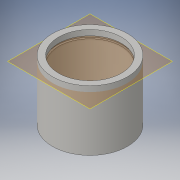
# Autodesk Inventor part: upper_arm_002
Saved by Autodesk Inventor 2016 SP1 (Build 200210100, 210)
## iProperties
Created: 2016-06-15
Part Number: upper_arm_002
Material: Generic
Document SubType Name: Modeling
Designer: asvsf
Density: 1 g/cm^3
Appearance: Default
Author: asvsf
Autodesk Inventor part; units mm, degrees
ref_plane "YZ Plane" through (0, 0, 0) normal (1, 0, 0) x (0, 1, 0)
ref_plane "XZ Plane" through (0, 0, 0) normal (0, 1, 0) x (-1, 0, 0)
ref_plane "XY Plane" through (0, 0, 0) normal (0, 0, 1) x (1, 0, 0)
sketch "Sketch1" plane through (0, 0, 0) normal (0, 1, 0) x (-1, 0, 0)
  circle A0 centre (0, 0) radius 31
  circle A1 centre (0, 0) radius 26
  dimension "d0" = 62
  dimension "d1" = 52
  constraints: 2 centre point, 2 coincident
  measures "d0" diameter of A0
  measures "d1" diameter of A1
extrude "Extrusion1" add sketch "Sketch1" along normal mid plane 50
ref_plane "Work Plane1" through (0, 20.5, 0) normal (0, 1, 0) x (1, 0, 0)
sketch "Sketch2" plane through (0, 20.5, 0) normal (0, 1, 0) x (1, 0, 0)
  circle A0 centre (0, 0) radius 27.5
  dimension "d5" = 55
  constraints: 1 centre point, 1 coincident
  measures "d5" diameter of A0
extrude "Extrusion2" cut sketch "Sketch2" against normal blind 2.15
mirror "Mirror1" about plane through (0, 0, 0) normal (0, 1, 0) of "Extrusion2"
body "Solid1"
